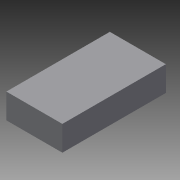
# Autodesk Inventor part: powerSupply
Saved by Autodesk Inventor 2013 (Build 170138000, 138)
## iProperties
Created: 2013-01-07
Part Number: powerSupply
Material: Generic
Document SubType Name: Modeling
Designer: james.eddlestone
Density: 1 g/cm^3
Author: james.eddlestone
Autodesk Inventor part; units mm, degrees
ref_plane "YZ Plane" through (0, 0, 0) normal (1, 0, 0) x (0, 1, 0)
ref_plane "XZ Plane" through (0, 0, 0) normal (0, 1, 0) x (-1, 0, 0)
ref_plane "XY Plane" through (0, 0, 0) normal (0, 0, 1) x (1, 0, 0)
sketch "Sketch1" plane through (0, 0, 0) normal (0, 0, 1) x (1, 0, 0)
  line L0 (0, 0) -> (114.3, 0)
  line L1 (114.3, 0) -> (114.3, 50.8)
  line L2 (114.3, 50.8) -> (0, 50.8)
  line L3 (0, 50.8) -> (0, 0)
  dimension "d0" = 114.3
  dimension "d1" = 50.8
  constraints: 8 end point, 2 parallel, 1 horizontal, 1 perpendicular
  measures "d0" distance of L2.end L1.end
  measures "d1" distance of L1.end L0.end
extrude "Extrusion1" add sketch "Sketch1" against normal blind 211.1375
sketch "Sketch2" plane through (0, 0, -211.1375) normal (0, 0, -1) x (-1, 0, 0)
  line L0 (-114.3, 0) -> (0, 0) projected
  line L1 (0, 0) -> (0, 50.8) projected
  line L2 (0, 50.8) -> (-114.3, 50.8) projected
  line L3 (-114.3, 50.8) -> (-114.3, 0) projected
  line L4 (-3.175, 7.9375) -> (-92.075, 7.9375)
  line L5 (-92.075, 7.9375) -> (-92.075, 25.4)
  line L6 (-92.075, 25.4) -> (-3.175, 25.4)
  line L7 (-3.175, 25.4) -> (-3.175, 7.9375)
  line L8 (-82.55, 25.4) -> (-80.9625, 25.4)
  line L9 (-80.9625, 25.4) -> (-80.9625, 7.9375)
  line L10 (-80.9625, 7.9375) -> (-82.55, 7.9375)
  line L11 (-82.55, 7.9375) -> (-82.55, 25.4)
  line L12 (-73.025, 25.4) -> (-71.4375, 25.4)
  line L13 (-71.4375, 25.4) -> (-71.4375, 7.9375)
  line L14 (-71.4375, 7.9375) -> (-73.025, 7.9375)
  line L15 (-73.025, 7.9375) -> (-73.025, 25.4)
  line L16 (-63.5, 25.4) -> (-61.9125, 25.4)
  line L17 (-61.9125, 25.4) -> (-61.9125, 7.9375)
  line L18 (-61.9125, 7.9375) -> (-63.5, 7.9375)
  line L19 (-63.5, 7.9375) -> (-63.5, 25.4)
  line L20 (-53.975, 25.4) -> (-52.3875, 25.4)
  line L21 (-52.3875, 25.4) -> (-52.3875, 7.9375)
  line L22 (-52.3875, 7.9375) -> (-53.975, 7.9375)
  line L23 (-53.975, 7.9375) -> (-53.975, 25.4)
  line L24 (-44.45, 25.4) -> (-42.8625, 25.4)
  line L25 (-42.8625, 25.4) -> (-42.8625, 7.9375)
  line L26 (-42.8625, 7.9375) -> (-44.45, 7.9375)
  line L27 (-44.45, 7.9375) -> (-44.45, 25.4)
  line L28 (-34.925, 25.4) -> (-33.3375, 25.4)
  line L29 (-33.3375, 25.4) -> (-33.3375, 7.9375)
  line L30 (-33.3375, 7.9375) -> (-34.925, 7.9375)
  line L31 (-34.925, 7.9375) -> (-34.925, 25.4)
  line L32 (-25.4, 25.4) -> (-23.8125, 25.4)
  line L33 (-23.8125, 25.4) -> (-23.8125, 7.9375)
  line L34 (-23.8125, 7.9375) -> (-25.4, 7.9375)
  line L35 (-25.4, 7.9375) -> (-25.4, 25.4)
  line L36 (-15.875, 25.4) -> (-14.2875, 25.4)
  line L37 (-14.2875, 25.4) -> (-14.2875, 7.9375)
  line L38 (-14.2875, 7.9375) -> (-15.875, 7.9375)
  line L39 (-15.875, 7.9375) -> (-15.875, 25.4)
  line L40 (-4.7625, 25.4) -> (-3.175, 25.4)
  line L41 (-3.175, 25.4) -> (-3.175, 7.9375)
  line L42 (-3.175, 7.9375) -> (-4.7625, 7.9375)
  line L43 (-4.7625, 7.9375) -> (-4.7625, 25.4)
  line L44 (-90.4875, 25.4) -> (-92.075, 25.4)
  line L45 (-92.075, 25.4) -> (-92.075, 7.9375)
  line L46 (-92.075, 7.9375) -> (-90.4875, 7.9375)
  line L47 (-90.4875, 7.9375) -> (-90.4875, 25.4)
  dimension "d4" = 3.175
  dimension "d5" = 7.9375
  dimension "d6" = 22.225
  dimension "d7" = 25.4
  dimension "d8" = 1.5875
  dimension "d9" = 7.9375
  dimension "d10" = 1.5875
  dimension "d11" = 7.9375
  dimension "d12" = 1.5875
  dimension "d13" = 7.9375
  dimension "d14" = 1.5875
  dimension "d15" = 7.9375
  dimension "d16" = 1.5875
  dimension "d17" = 7.9375
  dimension "d18" = 1.5875
  dimension "d19" = 1.5875
  dimension "d21" = 1.5875
  dimension "d23" = 1.5875
  dimension "d24" = 7.9375
  dimension "d25" = 1.5875
  dimension "d26" = 7.9375
  dimension "d27" = 7.9375
  constraints: 84 end point, 21 parallel, 10 horizontal, 10 perpendicular, 1 vertical, 24 other
  measures "d4" distance between parallel lines of L1 L7
  measures "d6" distance between parallel lines of L3 L5
  measures "d8" distance between parallel lines of L45 L47
  measures "d9" distance between parallel lines of L47 L11
  measures "d10" distance between parallel lines of L11 L9
  measures "d11" distance between parallel lines of L15 L9
  measures "d12" distance between parallel lines of L15 L13
  measures "d13" distance between parallel lines of L13 L19
  measures "d14" distance between parallel lines of L19 L17
  measures "d15" distance between parallel lines of L17 L23
  measures "d16" distance between parallel lines of L23 L21
  measures "d17" distance between parallel lines of L21 L27
  measures "d18" distance between parallel lines of L27 L25
  measures "d19" distance between parallel lines of L7 L43
  measures "d21" distance between parallel lines of L37 L39
  measures "d23" distance between parallel lines of L33 L35
  measures "d24" distance between parallel lines of L25 L31
  measures "d25" distance between parallel lines of L31 L29
  measures "d26" distance between parallel lines of L29 L35
  measures "d27" distance between parallel lines of L33 L39
extrude "Extrusion2" add sketch "Sketch2" along normal blind 15.875 contours L4 L43 L6 L7 | L4 L39 L6 L37 | L4 L35 L6 L33 | L4 L31 L6 L29 | L4 L27 L6 L25 | L4 L23 L6 L21 | L4 L19 L6 L17 | L4 L15 L6 L13 | L4 L11 L6 L9 | L4 L5 L6 L47
sketch "Sketch3" plane through (0, 0, -211.1375) normal (0, 0, -1) x (-1, 0, 0)
  line L0 (-71.4375, 7.9375) -> (-73.025, 7.9375) projected
  line L1 (-73.025, 7.9375) -> (-73.025, 25.4) projected
  line L2 (-52.3875, 7.9375) -> (-53.975, 7.9375) projected
  line L3 (-53.975, 7.9375) -> (-53.975, 25.4) projected
  line L4 (-33.3375, 7.9375) -> (-34.925, 7.9375) projected
  line L5 (-34.925, 7.9375) -> (-34.925, 25.4) projected
  line L6 (-23.8125, 7.9375) -> (-25.4, 7.9375) projected
  line L7 (-25.4, 7.9375) -> (-25.4, 25.4) projected
  line L8 (-14.2875, 7.9375) -> (-15.875, 7.9375) projected
  line L9 (-15.875, 7.9375) -> (-15.875, 25.4) projected
  line L10 (-42.8625, 7.9375) -> (-44.45, 7.9375) projected
  line L11 (-44.45, 7.9375) -> (-44.45, 25.4) projected
  line L12 (-61.9125, 7.9375) -> (-63.5, 7.9375) projected
  line L13 (-63.5, 7.9375) -> (-63.5, 25.4) projected
  line L14 (-80.9625, 7.9375) -> (-82.55, 7.9375) projected
  line L15 (-82.55, 7.9375) -> (-82.55, 25.4) projected
  line L16 (-92.075, 25.4) -> (-3.175, 25.4)
  line L17 (-3.175, 25.4) -> (-3.175, 7.9375)
  line L18 (-3.175, 7.9375) -> (-92.075, 7.9375)
  line L19 (-92.075, 7.9375) -> (-92.075, 25.4)
  line L20 (-90.4875, 7.9375) -> (-92.075, 7.9375)
  line L21 (-92.075, 7.9375) -> (-92.075, 25.4)
  line L22 (-92.075, 25.4) -> (-90.4875, 25.4)
  line L23 (-90.4875, 25.4) -> (-90.4875, 7.9375)
  line L24 (-82.55, 25.4) -> (-80.9625, 25.4)
  line L25 (-80.9625, 25.4) -> (-80.9625, 7.9375)
  line L26 (-80.9625, 7.9375) -> (-82.55, 7.9375)
  line L27 (-82.55, 7.9375) -> (-82.55, 25.4)
  line L28 (-73.025, 25.4) -> (-71.4375, 25.4)
  line L29 (-71.4375, 25.4) -> (-71.4375, 7.9375)
  line L30 (-71.4375, 7.9375) -> (-73.025, 7.9375)
  line L31 (-73.025, 7.9375) -> (-73.025, 25.4)
  line L32 (-63.5, 25.4) -> (-61.9125, 25.4)
  line L33 (-61.9125, 25.4) -> (-61.9125, 7.9375)
  line L34 (-61.9125, 7.9375) -> (-63.5, 7.9375)
  line L35 (-63.5, 7.9375) -> (-63.5, 25.4)
  line L36 (-53.975, 25.4) -> (-52.3875, 25.4)
  line L37 (-52.3875, 25.4) -> (-52.3875, 7.9375)
  line L38 (-52.3875, 7.9375) -> (-53.975, 7.9375)
  line L39 (-53.975, 7.9375) -> (-53.975, 25.4)
  line L40 (-44.45, 25.4) -> (-42.8625, 25.4)
  line L41 (-42.8625, 25.4) -> (-42.8625, 7.9375)
  line L42 (-42.8625, 7.9375) -> (-44.45, 7.9375)
  line L43 (-44.45, 7.9375) -> (-44.45, 25.4)
  line L44 (-34.925, 25.4) -> (-33.3375, 25.4)
  line L45 (-33.3375, 25.4) -> (-33.3375, 7.9375)
  line L46 (-33.3375, 7.9375) -> (-34.925, 7.9375)
  line L47 (-34.925, 7.9375) -> (-34.925, 25.4)
  line L48 (-25.4, 25.4) -> (-23.8125, 25.4)
  line L49 (-23.8125, 25.4) -> (-23.8125, 7.9375)
  line L50 (-23.8125, 7.9375) -> (-25.4, 7.9375)
  line L51 (-25.4, 7.9375) -> (-25.4, 25.4)
  line L52 (-15.875, 25.4) -> (-14.2875, 25.4)
  line L53 (-14.2875, 25.4) -> (-14.2875, 7.9375)
  line L54 (-14.2875, 7.9375) -> (-15.875, 7.9375)
  line L55 (-15.875, 7.9375) -> (-15.875, 25.4)
  line L56 (-4.7625, 25.4) -> (-3.175, 25.4)
  line L57 (-3.175, 25.4) -> (-3.175, 7.9375)
  line L58 (-3.175, 7.9375) -> (-4.7625, 7.9375)
  line L59 (-4.7625, 7.9375) -> (-4.7625, 25.4)
  constraints: 88 end point, 22 parallel, 11 horizontal, 11 perpendicular
extrude "Extrusion3" add sketch "Sketch3" along normal blind 6.35 contours L29 L16 L13 L18 | L18 L25 L16 L1 | L33 L16 L3 L18 | L18 L23 L16 L15 | L37 L16 L11 L18 | L41 L16 L5 L18 | L45 L16 L7 L18 | L49 L16 L9 L18 | L53 L16 L59 L18
body "Solid1"
